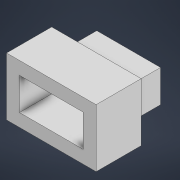
# Autodesk Inventor part: Cube_Holder_SB_V1_(71mm)
Saved by Autodesk Inventor 2022 (Build 260153000, 153)
## iProperties
Created: 2023-05-10
Part Number: Cube_Holder_SB_V1_(71mm)
Material: Generic
Document SubType Name: Modeling
Designer: Karl Spiteri
Density: 1 g/cm^3
Appearance: Default
Author: Karl Spiteri
Autodesk Inventor part; units mm, degrees
ref_plane "YZ Plane" through (0, 0, 0) normal (1, 0, 0) x (0, 1, 0)
ref_plane "XZ Plane" through (0, 0, 0) normal (0, 1, 0) x (-1, 0, 0)
ref_plane "XY Plane" through (0, 0, 0) normal (0, 0, 1) x (1, 0, 0)
sketch "Sketch5" plane through (0, 0, 0) normal (0, 0, 1) x (1, 0, 0)
  line L0 (0, 0) -> (-13.9, 0)
  line L1 (-13.9, 0) -> (-13.9, 9)
  line L2 (-13.9, 9) -> (0, 9)
  line L3 (0, 9) -> (0, 0)
  line L4 (-2, 2) -> (-11.9, 2)
  line L5 (-11.9, 2) -> (-11.9, 7)
  line L6 (-11.9, 7) -> (-2, 7)
  line L7 (-2, 7) -> (-2, 2)
  dimension "d67" = 13.9
  dimension "d68" = 9
  dimension "d69" = 9.9
  dimension "d70" = 5
  constraints: 16 end point, 4 parallel, 2 horizontal, 2 perpendicular
  measures "d67" distance of L1.end L2.end
  measures "d68" distance of L0.end L1.end
  measures "d69" distance of L5.end L6.end
  measures "d70" distance of L4.end L5.end
extrude "Extrusion8" add sketch "Sketch5" along normal blind 7 contours L0 L1 L2 L3 | L4 L5 L6 L7
sketch "Sketch6" plane through (0, 0, 7) normal (0, 0, 1) x (1, 0, 0)
  line L0 (-2, 2) -> (-11.9, 2)
  line L1 (-11.9, 2) -> (-11.9, 7)
  line L2 (-11.9, 7) -> (-2, 7)
  line L3 (-2, 7) -> (-2, 2)
  point P0 (0, 0)
  dimension "d73" = 9.9
  dimension "d74" = 5
  constraints: 8 end point, 2 parallel, 1 horizontal, 1 perpendicular
  measures "d73" distance of L1.end L2.end
  measures "d74" distance of L0.end L1.end
extrude "Extrusion9" cut sketch "Sketch6" against normal blind 5
sketch "Sketch7" plane through (0, 0, 0) normal (0, 0, -1) x (-1, 0, 0)
  line L0 (2, 2) -> (11.9, 2)
  line L1 (11.9, 2) -> (11.9, 7)
  line L2 (11.9, 7) -> (2, 7)
  line L3 (2, 7) -> (2, 2)
  point P0 (0, 0)
  dimension "d77" = 9.9
  dimension "d78" = 5
  constraints: 8 end point, 2 parallel, 1 horizontal, 1 perpendicular
  measures "d77" distance of L2.end L1.end
  measures "d78" distance of L1.end L0.end
extrude "Extrusion10" add sketch "Sketch7" along normal blind 5
body "Solid7"
